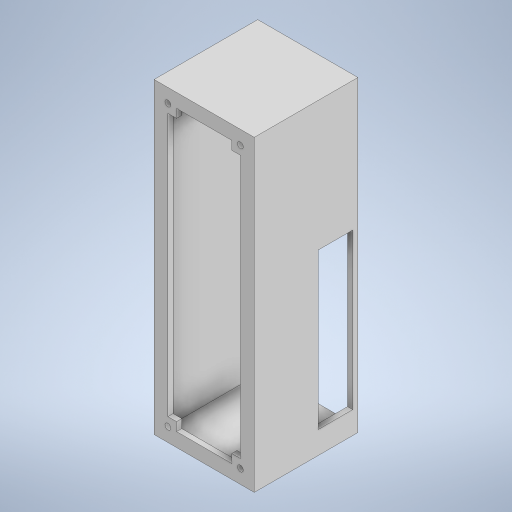
# Autodesk Inventor part: port side
Saved by Autodesk Inventor 2023 (Build 270158030, 158C)
## iProperties
Created: 2023-03-06
Part Number: port side
Material: Generic
Document SubType Name: Modeling
Designer: fatih
Density: 1 g/cm^3
Appearance: Default
Author: fatih
Autodesk Inventor part; units mm, degrees
ref_plane "YZ Plane" through (0, 0, 0) normal (1, 0, 0) x (0, 1, 0)
ref_plane "XZ Plane" through (0, 0, 0) normal (0, 1, 0) x (-1, 0, 0)
ref_plane "XY Plane" through (0, 0, 0) normal (0, 0, 1) x (1, 0, 0)
sketch "Sketch1" plane through (0, 0, 0) normal (0, 0, 1) x (1, 0, 0)
  line L0 (0, 0) -> (58, 0)
  line L1 (58, 0) -> (58, 178)
  line L2 (58, 178) -> (0, 178)
  line L3 (0, 178) -> (0, 0)
  dimension "d0" = 58
  dimension "d1" = 178
  constraints: 8 end point, 2 parallel, 1 horizontal, 1 perpendicular
  measures "d0" distance of L1.end L2.end
  measures "d1" distance of L2.end L0.start
extrude "Extrusion1" add sketch "Sketch1" along normal blind 60
shell "Shell1" thickness 3 removed faces 1 at (19.3333, 118.6667, 0)
sketch "Sketch2" plane through (0, 0, 60) normal (0, 0, 1) x (1, 0, 0)
  line L0 (3, 3) -> (55, 3) projected
  line L1 (3, 3) -> (8, 3)
  line L2 (8, 3) -> (8, 6.3)
  line L3 (55, 3) -> (55, 175) projected
  line L4 (55, 175) -> (55, 170)
  line L5 (55, 170) -> (51.7, 170)
  line L6 (48.3, 170) -> (9.7, 170)
  line L7 (8, 168.3) -> (8, 9.7)
  line L8 (9.7, 8) -> (48.3, 8)
  line L9 (50, 9.7) -> (50, 168.3)
  circle A0 centre (8, 8) radius 1.7
  line L10 (9.7, 8) -> (13, 8)
  line L11 (8, 9.7) -> (8, 13)
  line L12 (8, 13) -> (13, 13)
  line L13 (13, 13) -> (13, 8)
  line L14 (29, 8) -> (29, 9.7)
  circle A1 centre (50, 8) radius 1.7
  line L15 (48.3, 8) -> (45, 8)
  line L16 (50, 9.7) -> (50, 13)
  line L17 (50, 13) -> (45, 13)
  line L18 (45, 13) -> (45, 8)
  line L19 (50, 89) -> (45, 89)
  circle A2 centre (8, 170) radius 1.7
  line L20 (9.7, 170) -> (13, 170)
  line L21 (8, 168.3) -> (8, 165)
  line L22 (8, 165) -> (13, 165)
  line L23 (13, 165) -> (13, 170)
  circle A3 centre (50, 170) radius 1.7
  line L24 (48.3, 170) -> (45, 170)
  line L25 (50, 168.3) -> (50, 165)
  line L26 (45, 165) -> (45, 170)
  line L27 (50, 165) -> (45, 165)
  point P0 (0, 0)
  point P1 (58, 0)
  point P2 (58, 178)
  point P3 (0, 178)
  point P4 (50, 6.3)
  point P5 (8, 171.7)
  point P6 (50, 171.7)
  dimension "d29" = 5
  dimension "d31" = 5
  dimension "d32" = 5
  dimension "d33" = 3.4
  dimension "d34" = 3.3
  dimension "d35" = 3.3
  constraints: 52 end point, 18 symmetric about line, 13 point on circle, 6 perpendicular, 4 centre point, 4 point on line, 2 horizontal, 2 midpoint, 2 parallel, 3 other
  measures "d29" distance of L0.start L1.end
  measures "d31" distance of L3.end L4.end
  measures "d32" distance of L4.end A3.centre
  measures "d33" diameter of A0
  measures "d34" distance of L8.start L10.end
  measures "d35" distance of L7.end L11.end
extrude "Extrusion4" cut sketch "Sketch2" against normal blind 3 contours A0 | A3 | L7 L22 L23 L6 L26 L27 L9 L17 L18 L8 L13 L12 | A2 | A1
sketch "Sketch4" plane through (58, 0, 0) normal (1, 0, 0) x (0, 0, -1)
  line L0 (0, 3) -> (-57, 3) projected
  line L1 (0, 3) -> (-3, 3)
  line L2 (-3, 3) -> (-23, 3)
  line L3 (-23, 3) -> (-23, 103)
  line L4 (-23, 103) -> (-3, 103)
  line L5 (-3, 103) -> (-3, 3)
  line L6 (-23, 3) -> (-23, 13)
  line L7 (-23, 13) -> (-3, 13)
  point P0 (0, 0)
  dimension "d38" = 3
  dimension "d39" = 20
  dimension "d40" = 100
  dimension "d41" = 10
  constraints: 14 end point, 3 point on line, 2 parallel, 2 perpendicular, 1 horizontal
  measures "d38" distance of L0.start L1.end
  measures "d39" distance of L3.end L4.end
  measures "d40" distance of L2.end L3.end
  measures "d41" distance of L2.end L6.end
extrude "Extrusion5" cut sketch "Sketch4" against normal blind 4 contours L7 L3 L4 L5
body "Solid1"
